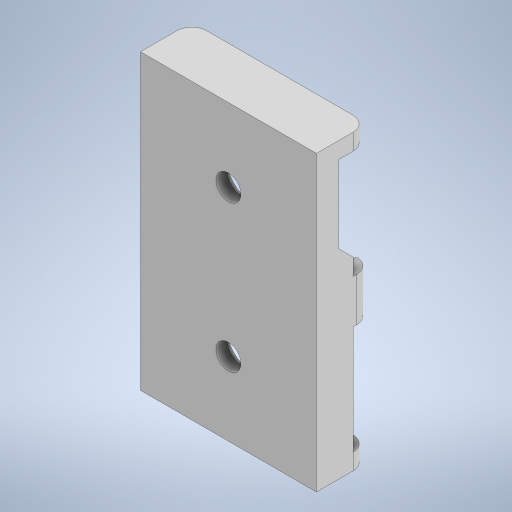
# Autodesk Inventor part: Halter_Treiber_LED
Saved by Autodesk Inventor 2024 (Build 280153000, 153)
## iProperties
Created: 2024-10-16
Part Number: Halter_Treiber_LED
Material: Generisch
Document SubType Name: Modeling
Designer: month
Density: 1 g/cm^3
Appearance: Vorgabe
Author: month
Autodesk Inventor part; units mm, degrees
ref_plane "YZ Plane" through (0, 0, 0) normal (1, 0, 0) x (0, 1, 0)
ref_plane "XZ Plane" through (0, 0, 0) normal (0, 1, 0) x (-1, 0, 0)
ref_plane "XY Plane" through (0, 0, 0) normal (0, 0, 1) x (1, 0, 0)
sketch "Skizze1" plane through (0, 0, 0) normal (0, 1, 0) x (-1, 0, 0)
  line L0 (0, 0) -> (24, 0)
  line L1 (24, 0) -> (24, -40)
  line L2 (24, -40) -> (0, -40)
  line L3 (0, -40) -> (0, 0)
  dimension "d0" = 40
  dimension "d1" = 24
  constraints: 8 end point, 2 parallel, 1 horizontal, 1 perpendicular
  measures "d0" distance of L0.end L1.end
  measures "d1" distance of L1.end L2.end
extrude "Extrusion1" add sketch "Skizze1" along normal blind 3
sketch "Skizze2" plane through (0, 3, 0) normal (0, 1, 0) x (1, 0, 0)
  line L0 (-24, 40) -> (-24, 0) projected
  line L1 (0, 0) -> (0, 40) projected
  line L2 (-24, 0) -> (0, 0)
  line L3 (0, 0) -> (0, 2.25)
  line L4 (0, 2.25) -> (-24, 2.25)
  line L5 (-24, 2.25) -> (-24, 0)
  line L6 (0, 40) -> (-24, 40) projected
  line L7 (-24, 40) -> (0, 40)
  line L8 (0, 40) -> (0, 37.75)
  line L9 (0, 37.75) -> (-24, 37.75)
  line L10 (-24, 37.75) -> (-24, 40)
  dimension "d4" = 2.25
  dimension "d5" = 2.25
  constraints: 16 end point, 4 parallel, 2 horizontal, 2 perpendicular, 2 point on line
  measures "d4" distance between parallel lines of L4 L2
  measures "d5" distance between parallel lines of L9 L6
extrude "Extrusion2" add sketch "Skizze2" along normal blind 4 contours L6 L1 L9 L0 | L4 L1 L2 L0
sketch "Skizze4" plane through (0, 3, 0) normal (0, 1, 0) x (1, 0, 0)
  line L0 (0, 2.25) -> (-24, 2.25) projected
  line L1 (0, 2.25) -> (-1.8184, 2.25)
  line L2 (0, 37.75) -> (-1.8184, 37.75)
  line L3 (-24.0183, 2.25) -> (-21.7244, 2.25)
  line L4 (-24, 37.75) -> (-21.1801, 37.75)
  line L5 (0, 37.75) -> (-4, 37.75)
  line L6 (-4, 37.75) -> (-4, 12.75)
  line L7 (-4, 12.75) -> (0, 12.75)
  line L8 (0, 12.75) -> (0, 37.75)
  line L9 (-24, 37.75) -> (-24, 2.25) projected
  line L10 (-24, 10) -> (-20, 10)
  line L11 (-20, 10) -> (-20, 30)
  line L12 (-20, 30) -> (-24, 30)
  line L13 (-24, 30) -> (-24, 10)
  line L14 (-24, 0) -> (0, 0) projected
  dimension "d25" = 25
  dimension "d26" = 4
  dimension "d27" = 4
  dimension "d29" = 20
  dimension "d30" = 10
  constraints: 24 end point, 6 horizontal, 4 parallel, 4 point on line, 2 perpendicular
  measures "d25" distance of L7.end L2.start
  measures "d26" distance of L6.end L7.end
  measures "d27" distance of L10.start L10.end
  measures "d29" distance between parallel lines of L10 L12
  measures "d30" distance between parallel lines of L14 L10
extrude "Extrusion4" add sketch "Skizze4" along normal blind 2
sketch "Skizze5" plane through (0, 5, 0) normal (0, 1, 0) x (1, 0, 0)
  line L0 (-24, 30) -> (-24, 10) projected
  line L1 (-24, 20) -> (0, 20)
  line L2 (0, 0) -> (0, 40) projected
  line L3 (-24, 18.5) -> (-22.2, 18.5)
  line L4 (-22.2, 18.5) -> (-22.2, 21.5)
  line L5 (-22.2, 21.5) -> (-24, 21.5)
  line L6 (-24, 21.5) -> (-24, 18.5)
  line L7 (0, 17) -> (-1.8, 17)
  line L8 (-1.8, 17) -> (-1.8, 23)
  line L9 (-1.8, 23) -> (0, 23)
  line L10 (0, 23) -> (0, 17)
  point P0 (-23.1, 18.5)
  point P1 (0, 23)
  dimension "d33" = 3
  dimension "d34" = 1.8
  dimension "d35" = 1.8
  dimension "d36" = 6
  constraints: 18 end point, 4 parallel, 3 midpoint, 2 horizontal, 2 perpendicular, 2 point on line, 2 other
  measures "d33" distance from line of point (-23.1, 18.5) L5
  measures "d34" distance between parallel lines of L0 L4
  measures "d35" distance of L8.end L9.end
  measures "d36" distance between parallel lines of L7 L9
extrude "Extrusion5" add sketch "Skizze5" along normal blind 2.5
sketch "Skizze6" plane through (-1.8, 5, -23) normal (-1, 0, 0) x (0, 0, 1)
  line L0 (0, 0) -> (0, 2.5) projected
  line L1 (6, 0) -> (6, 2.5) projected
  line L2 (0, 2.5) -> (6, 2.5)
  line L3 (6, 2.5) -> (6, 1.5)
  line L4 (6, 1.5) -> (0, 1.5)
  line L5 (0, 1.5) -> (0, 2.5)
  point P0 (23, -5)
  point P1 (0, 1.5)
  dimension "d39" = 1
  constraints: 8 end point, 2 parallel, 1 horizontal, 1 perpendicular, 1 point on line
  measures "d39" distance between parallel lines of L2 L4
extrude "Extrusion6" add sketch "Skizze6" along normal blind 1
sketch "Skizze7" plane through (0, 5, -23) normal (0, 0, -1) x (-1, 0, 0)
  line L0 (2.8, 2.5) -> (2.8, 1.5) projected
  line L1 (2.8, 1.5) -> (1.8, 2.5)
  line L2 (0, 2.5) -> (2.8, 2.5) projected
  line L3 (1.8, 2.5) -> (2.8, 2.5)
  line L4 (2.8, 2.5) -> (2.8, 1.5)
  point P0 (0, -5)
  dimension "d42" = 1
  dimension "d43" = 1
  constraints: 6 end point, 2 point on line, 1 horizontal, 1 perpendicular
  measures "d42" distance of L0.start L1.end
  measures "d43" distance of L1.start L0.start
extrude "Extrusion7" cut sketch "Skizze7" against normal blind 10
sketch "Skizze9" plane through (-22.2, 5, -18.5) normal (1, 0, 0) x (0, 0, -1)
  line L0 (0, 0) -> (0, 2.5) projected
  line L1 (3, 0) -> (3, 2.5) projected
  line L2 (0, 2.5) -> (3, 2.5)
  line L3 (3, 2.5) -> (3, 1.5)
  line L4 (3, 1.5) -> (0, 1.5)
  line L5 (0, 1.5) -> (0, 2.5)
  line L6 (3, 0) -> (0, 0) projected
  point P0 (-18.5, -5)
  point P1 (0, 1.5)
  dimension "d46" = 1.5
  constraints: 8 end point, 2 parallel, 1 horizontal, 1 perpendicular, 1 point on line
  measures "d46" distance between parallel lines of L6 L4
extrude "Extrusion8" add sketch "Skizze9" along normal blind 0.5 contours L0 L2 L1 L4
sketch "Skizze11" plane through (-22.2, 5, -21.5) normal (0, 0, -1) x (-1, 0, 0)
  line L0 (-0.5, 2.5) -> (-0.5, 1.5)
  line L1 (-0.5, 1.5) -> (0, 2.5)
  line L2 (1.8, 2.5) -> (-0.5, 2.5) projected
  line L3 (-0.5, 1.5) -> (-0.5, 2.5) projected
  line L4 (-0.5, 2.5) -> (0, 2.5)
  point P0 (-22.2, -5)
  dimension "d49" = 0.5
  constraints: 6 end point, 1 collinear, 1 point on line
  measures "d49" distance of L0.start L1.end
extrude "Extrusion9" cut sketch "Skizze11" against normal blind 10
chamfer "Fasen1" distance 2 angle 45 3 edges at (-22, 5, -30) (-22, 5, -10) (-2, 5, -12.75)
fillet "Rundung1" radius 2 6 edges at (0, 7.5, -20) (-24, 7.5, -20) (-24, 7, -1.125) (0, 7, -1.125) (-24, 7, -38.875) (0, 7, -38.875)
sketch "Skizze12" plane through (0, 3, 0) normal (0, 1, 0) x (1, 0, 0)
  line L0 (-24, 0) -> (0, 0) projected
  line L1 (-12, 0) -> (-12, 40)
  line L2 (0, 40) -> (-24, 40) projected
  circle A0 centre (-12, 10) radius 2
  circle A1 centre (-12, 30) radius 2
  line L3 (-24, 40) -> (-24, 0) projected
  line L4 (-24, 20) -> (0, 20) construction
  line L5 (0, 17) -> (0, 23) projected
  dimension "d56" = 4
  dimension "d57" = 4
  dimension "d58" = 20
  constraints: 4 end point, 4 midpoint, 2 centre point, 2 point on line, 1 symmetric about line
  measures "d56" diameter of A0
  measures "d57" diameter of A1
  measures "d58" distance of A0.centre A1.centre
hole "Bohrung1" at (-12, 3, -10) at (-12, 3, -30) direction (0, -1, 0) diameter 3.4 depth 8.8 tip angle 118 countersink diameter 6.3 countersink angle 90 clearance for "Flachkopfsenkschraube ISO 2009/7046" size "M3" standard "ISO"
